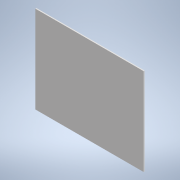
# Autodesk Inventor part: filter1
Saved by Autodesk Inventor 2022 (Build 260153000, 153)
## iProperties
Created: 2024-07-15
Part Number: filter1
Material: Типовые
Document SubType Name: Modeling
Designer: Капустяник Андрей
Density: 1 g/cm^3
Appearance: По умолчанию
Author: Капустяник Андрей
Autodesk Inventor part; units mm, degrees
ref_plane "YZ Plane" through (0, 0, 0) normal (1, 0, 0) x (0, 1, 0)
ref_plane "XZ Plane" through (0, 0, 0) normal (0, 1, 0) x (-1, 0, 0)
ref_plane "XY Plane" through (0, 0, 0) normal (0, 0, 1) x (1, 0, 0)
sketch "Эскиз1" plane through (0, 0, 0) normal (0, 0, 1) x (1, 0, 0)
  line L0 (-50, -10.7689) -> (0.7689, 40) projected
  line L1 (-50, -3.56) -> (-50, -10.7689) projected
  line L2 (-6.44, 40) -> (-50, -3.56) projected
  line L3 (0.7689, 40) -> (-6.44, 40) projected
  line L4 (-22.1111, -40) -> (50, 32.1111) projected
  line L5 (-29.32, -40) -> (-22.1111, -40) projected
  line L6 (50, 39.32) -> (-29.32, -40) projected
  line L7 (50, 32.1111) -> (50, 39.32) projected
  line L8 (50, -17.8) -> (27.8, -40) projected
  line L9 (50, -25) -> (50, -17.8) projected
  line L10 (35, -40) -> (50, -25) projected
  line L11 (27.8, -40) -> (35, -40) projected
  line L12 (-7.8311, -40) -> (50, 17.8311) projected
  line L13 (-15.04, -40) -> (-7.8311, -40) projected
  line L14 (50, 25.04) -> (-15.04, -40) projected
  line L15 (50, 17.8311) -> (50, 25.04) projected
  line L16 (-50, -25.0489) -> (15.0489, 40) projected
  line L17 (-50, -17.84) -> (-50, -25.0489) projected
  line L18 (7.84, 40) -> (-50, -17.84) projected
  line L19 (15.0489, 40) -> (7.84, 40) projected
  line L20 (-50, 3.5111) -> (-13.5111, 40) projected
  line L21 (-50, 10.72) -> (-50, 3.5111) projected
  line L22 (-20.72, 40) -> (-50, 10.72) projected
  line L23 (-13.5111, 40) -> (-20.72, 40) projected
  line L24 (-36.3911, -40) -> (43.6089, 40) projected
  line L25 (-43.6, -40) -> (-36.3911, -40) projected
  line L26 (36.4, 40) -> (-43.6, -40) projected
  line L27 (43.6089, 40) -> (36.4, 40) projected
  line L28 (20.7289, -40) -> (50, -10.7289) projected
  line L29 (13.52, -40) -> (20.7289, -40) projected
  line L30 (50, -3.52) -> (13.52, -40) projected
  line L31 (50, -10.7289) -> (50, -3.52) projected
  line L32 (6.4489, -40) -> (50, 3.5511) projected
  line L33 (-0.76, -40) -> (6.4489, -40) projected
  line L34 (50, 10.76) -> (-0.76, -40) projected
  line L35 (50, 3.5511) -> (50, 10.76) projected
  line L36 (-50, -39.3289) -> (29.3289, 40) projected
  line L37 (-50, -32.12) -> (-50, -39.3289) projected
  line L38 (22.12, 40) -> (-50, -32.12) projected
  line L39 (29.3289, 40) -> (22.12, 40) projected
  line L40 (-50, 17.7911) -> (-27.7911, 40) projected
  line L41 (-50, 25) -> (-50, 17.7911) projected
  line L42 (-35, 40) -> (-50, 25) projected
  line L43 (-27.7911, 40) -> (-35, 40) projected
  line L44 (52, -42) -> (-52, -42) projected
  line L45 (52, 42) -> (52, -42) projected
  line L46 (-52, 42) -> (52, 42) projected
  line L47 (-52, -42) -> (-52, 42) projected
  line L48 (51.6, 41.6) -> (51.6, -41.6)
  line L49 (51.6, -41.6) -> (-51.6, -41.6)
  line L50 (-51.6, -41.6) -> (-51.6, 41.6)
  line L51 (-51.6, 41.6) -> (51.6, 41.6)
  point P0 (0, 0)
  dimension "d0" = 0.4
  constraints: 8 end point, 3 other
  measures "d0" distance between parallel lines of L46 L51
extrude "Выдавливание1" add sketch "Эскиз1" along normal blind 1 contours L1 L2 L3 L0 | L5 L6 L7 L4 | L9 L10 L11 L8 | L13 L14 L15 L12 | L17 L18 L19 L16 | L21 L22 L23 L20 | L25 L26 L27 L24 | L29 L30 L31 L28 | L33 L34 L35 L32 | L37 L38 L39 L36 | L41 L42 L43 L40 | L48 L49 L50 L51
